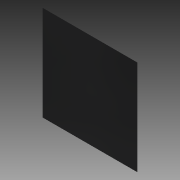
# Autodesk Inventor part: Square_Velostat
Saved by Autodesk Inventor 2014 SP1 (Build 180222100, 222)
## iProperties
Created: 2014-01-12
Part Number: Square_Velostat
Material: Rubber
Document SubType Name: Modeling
Designer: tuleu
Density: 0.93 g/cm^3
Appearance: Rubber - Black - Version 1.1
Author: tuleu
Autodesk Inventor part; units mm, degrees
ref_plane "YZ Plane" through (0, 0, 0) normal (1, 0, 0) x (0, 1, 0)
ref_plane "XZ Plane" through (0, 0, 0) normal (0, 1, 0) x (-1, 0, 0)
ref_plane "XY Plane" through (0, 0, 0) normal (0, 0, 1) x (1, 0, 0)
sketch "Sketch1" plane through (0, 0, 0) normal (0, 1, 0) x (-1, 0, 0)
  line L0 (-75, -75) -> (75, -75)
  line L1 (75, -75) -> (75, 75)
  line L2 (75, 75) -> (-75, 75)
  line L3 (-75, 75) -> (-75, -75)
  line L4 (0, -75) -> (0, 75) construction
  line L5 (75, 0) -> (-75, 0) construction
  point P0 (0, 0)
  dimension "d0" = 150
  constraints: 12 end point, 6 midpoint, 2 parallel, 2 perpendicular, 1 horizontal
  measures "d0" distance of L0.start L0.end
extrude "Extrusion1" add sketch "Sketch1" along normal mid plane 0.01
body "Solid1"
